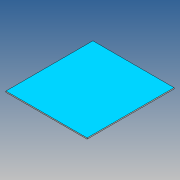
# Autodesk Inventor part: botonera
Saved by Autodesk Inventor 2017 (Build 210142000, 142)
## iProperties
Part Number: botonera
Material: Genérico
Document SubType Name: Modeling
Designer: Leo
Density: 1 g/cm^3
Appearance: Valor por defecto
Author: Leo
Autodesk Inventor part; units mm, degrees
ref_plane "YZ Plane" through (0, 0, 0) normal (1, 0, 0) x (0, 1, 0)
ref_plane "XZ Plane" through (0, 0, 0) normal (0, 1, 0) x (-1, 0, 0)
ref_plane "XY Plane" through (0, 0, 0) normal (0, 0, 1) x (1, 0, 0)
sketch "Boceto1" plane through (0, 0, 0) normal (0, 0, 1) x (1, 0, 0)
  line L0 (-35, 37.5) -> (35, 37.5)
  line L1 (35, 37.5) -> (35, -37.5)
  line L2 (35, -37.5) -> (-35, -37.5)
  line L3 (-35, -37.5) -> (-35, 37.5)
  point P0 (0, 0)
  point P1 (-35, 0)
  point P2 (0, 37.5)
  dimension "d0" = 70
  dimension "d1" = 75
  constraints: 8 end point, 2 midpoint, 2 parallel, 1 horizontal, 1 horizontal alignment, 1 perpendicular, 1 vertical alignment
  measures "d0" distance of L0.start L0.end
  measures "d1" distance of L2.end L0.start
extrude "Extrusión1" add sketch "Boceto1" along normal blind 1
